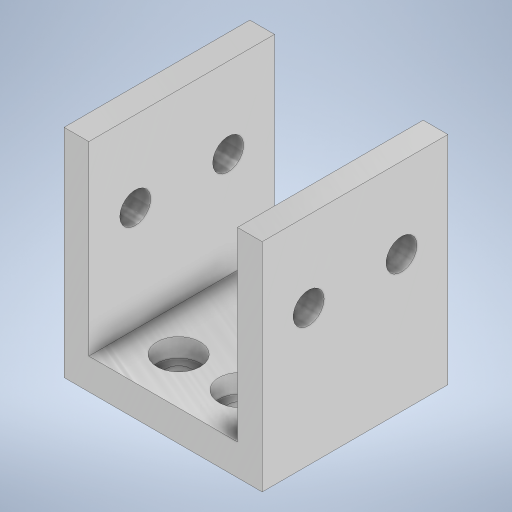
# Autodesk Inventor part: Suporte braço 2.0
Saved by Autodesk Inventor 2023.2 (Build 272271030, 271C)
## iProperties
Created: 2023-03-25
Part Number: Suporte braço 2.0
Material: Aço galvanizado
Document SubType Name: Sheet Metal
Designer: Mateus
Density: 7.85 g/cm^3
Sheet Metal Rule: Padrão_mm
Appearance: Usinado - Alumínio
Mass: 88.7745 g
Surface Area: 69.1531 cm^2
Volume: 11.3088 cm^3
Author: Mateus
Autodesk Inventor part; units mm, degrees
ref_plane "YZ Plane" through (0, 0, 0) normal (1, 0, 0) x (0, 1, 0)
ref_plane "XZ Plane" through (0, 0, 0) normal (0, 1, 0) x (-1, 0, 0)
ref_plane "XY Plane" through (0, 0, 0) normal (0, 0, 1) x (1, 0, 0)
sketch "Esboço1" plane through (0, 0, 0) normal (0, 1, 0) x (-1, 0, 0)
  line L0 (0, 0) -> (32, 0)
  line L1 (32, 0) -> (32, -30)
  line L2 (32, -30) -> (0, -30)
  line L3 (0, -30) -> (0, 0)
  dimension "d0" = 32
  dimension "d1" = 30
  constraints: 8 end point, 2 parallel, 1 horizontal, 1 perpendicular
  measures "d0" distance of L1.end L2.end
  measures "d1" distance of L0.end L1.end
extrude "Extrusion1" add sketch "Esboço1" along normal blind 5
sketch "Sketch4" plane through (0, 5, 0) normal (0, 1, 0) x (1, 0, 0)
  line L0 (0, 30) -> (-32, 30) projected
  line L1 (-32, 30) -> (-28, 30)
  line L2 (-28, 30) -> (-28, 0)
  line L3 (-28, 0) -> (-32, 0)
  line L4 (-32, 0) -> (-32, 30)
  line L5 (-4, 30) -> (0, 30)
  line L6 (0, 30) -> (0, 0)
  line L7 (0, 0) -> (-4, 0)
  line L8 (-4, 0) -> (-4, 30)
  dimension "d26" = 4
  dimension "d27" = 4
  constraints: 16 end point, 5 parallel, 2 horizontal, 2 perpendicular
  measures "d26" distance of L0.end L1.end
  measures "d27" distance of L0.start L5.start
extrude "Extrusion2" add sketch "Sketch4" along normal blind 30
sketch "Sketch5" plane through (0, 0, 0) normal (1, 0, 0) x (0, 0, -1)
  line L0 (0, 0) -> (0, 35) projected
  line L1 (30, 0) -> (30, 35) projected
  line L2 (0, 35) -> (30, 35) projected
  point P0 (7.5, 22)
  point P1 (22.5, 22)
  dimension "d30" = 7.5
  dimension "d31" = 7.5
  dimension "d32" = 13
  dimension "d33" = 13
  measures "d30" distance from line of L0 point (7.5, 22)
  measures "d31" distance from line of L1 point (22.5, 22)
  measures "d32" distance from line of L2 point (22.5, 22)
  measures "d33" distance from line of L2 point (7.5, 22)
hole "Hole2" at (0, 22, -7.5) at (0, 22, -22.5) direction (-1, 0, 0) diameter 5 end through all
sketch "Esboço6" plane through (0, 5, 0) normal (0, 1, 0) x (1, 0, 0)
  line L0 (-4, 30) -> (-28, 30) projected
  line L1 (-28, 0) -> (-28, 30) projected
  line L2 (-32, 30) -> (-32, 0) projected
  point P0 (0, 0)
  point P1 (-21, 22.5)
  point P2 (-11, 22.5)
  point P3 (-11, 7.5)
  point P4 (-21, 7.5)
  dimension "d41" = 10
  dimension "d42" = 10
  dimension "d43" = 15
  dimension "d44" = 15
  dimension "d45" = 24
  dimension "d46" = 7
  dimension "d47" = 0
  dimension "d48" = 30
  dimension "d49" = 7.5
  measures "d41" distance of point (-21, 22.5) point (-11, 22.5)
  measures "d42" distance of point (-11, 7.5) point (-21, 7.5)
  measures "d43" distance of point (-11, 22.5) point (-11, 7.5)
  measures "d44" distance of point (-21, 22.5) point (-21, 7.5)
  measures "d45" distance of L0.start L0.end
  measures "d46" distance from line of L1 point (-21, 22.5)
  measures "d47" vertical distance of point (-21, 7.5) point (-11, 7.5)
  measures "d48" distance of L1.start L0.end
  measures "d49" distance from line of L0 point (-21, 22.5)
hole "Furo3" at (-21, 5, -22.5) at (-11, 5, -22.5) at (-11, 5, -7.5) at (-21, 5, -7.5) direction (0, -1, 0) diameter 4 depth 5 tip angle 118 counterbore diameter 7 counterbore depth 3
equation "\"d31\" = d30"
equation "\"d33\" = d32"
equation "\"d39\" = Espessura"
equation "\"d46\" = -0.5 * d41 + 0.5 * d45"
equation "\"d49\" = -0.5 * d44 + 0.5 * d48"
equation "\"d55\" = Espessura"
equation "\"Raio_vergadura\" = Espessura"
equation "\"Largura_alívio_de_vergadura\" = Espessura"
equation "\"Profundidade_alívio_de_vergadura\" = 0.5 * Espessura"
equation "\"Raiodetransição\" = Raio_vergadura"
equation "\"Tamanho_de_raio_de_Jacobi\" = Raio_vergadura"
equation "\"TamanhoFolga\" = Espessura"
equation "\"Espessura\" = 5"
body "Solid2"
